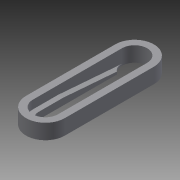
# Autodesk Inventor part: bed-holder
Saved by Autodesk Inventor 2015 (Build 190159000, 159)
## iProperties
Created: 2014-10-22
Part Number: bed-holder
Material: Generic
Document SubType Name: Modeling
Designer: caleb
Density: 1 g/cm^3
Appearance: Default
screw_diameter: 4.500 mm
screw_head_diameter: 7.500 mm
screw_head_clearance: 2.500 mm
wall: 2.000 mm
length: 38.000 mm
height: 4.500 mm
land_height: 2.000 mm
Author: caleb
Autodesk Inventor part; units mm, degrees
ref_plane "YZ Plane" through (0, 0, 0) normal (1, 0, 0) x (0, 1, 0)
ref_plane "XZ Plane" through (0, 0, 0) normal (0, 1, 0) x (-1, 0, 0)
ref_plane "XY Plane" through (0, 0, 0) normal (0, 0, 1) x (1, 0, 0)
sketch "Sketch6" plane through (0, 0, 0) normal (0, 0, 1) x (1, 0, 0)
  line L0 (0, 0) -> (0, -26.5) construction
  line L1 (-3.75, 0) -> (-3.75, -26.5)
  line L2 (3.75, -26.5) -> (3.75, 0)
  arc A0 (3.75, 0) -> (-3.75, 0) centre (0, 0) ccw
  arc A1 (-3.75, -26.5) -> (3.75, -26.5) centre (0, -26.5) ccw
  line L3 (5.75, 0) -> (5.75, -26.5)
  arc A2 (-5.75, -26.5) -> (5.75, -26.5) centre (0, -26.5) ccw
  line L4 (-5.75, -26.5) -> (-5.75, 0)
  arc A3 (5.75, 0) -> (-5.75, 0) centre (0, 0) ccw
  line L5 (0, 5.75) -> (0, -32.25) construction
  line L6 (0, 0) -> (0, -26.5) construction
  line L7 (-2.25, 0) -> (-2.25, -3)
  line L8 (2.25, -26.5) -> (2.25, -3)
  arc A4 (2.25, 0) -> (-2.25, 0) centre (0, 0) ccw
  arc A5 (-2.25, -26.5) -> (2.25, -26.5) centre (0, -26.5) ccw
  arc A6 (-3.75, 0) -> (3.75, 0) centre (0, 0) ccw
  line L9 (-2.25, -3) -> (-2.25, -26.5)
  line L10 (2.25, -3) -> (2.25, 0)
  point P0 (0, -13.25)
  point P1 (0, -13.25)
  dimension "d20" = 3.75
  dimension "d21" = 2
  dimension "d22" = 38
  dimension "d23" = 4.5
  constraints: 26 end point, 18 point on circle, 13 tangent, 7 centre point, 6 parallel, 2 midpoint, 1 collinear, 1 vertical, 3 other
  measures "d20" radius of A0
  measures "d21" distance between parallel lines of L3 L2
  measures "d22" distance of L5.start L5.end
  measures "d23" distance between parallel lines of L8 L7
extrude "Extrusion7" add sketch "Sketch6" along normal blind 4.5
sketch "Sketch7" plane through (0, 0, 0) normal (1, 0, 0) x (0, 1, 0)
  line L0 (0, 0.5) -> (-19, 2) construction
  line L1 (-19, 2) -> (-19, 0) construction
  point P0 (0, 0)
  point P1 (-26.5, 0)
  dimension "d28" = 7.5
  dimension "d29" = 2
  dimension "d30" = 0.5
  constraints: 4 end point, 1 horizontal alignment, 1 vertical, 1 vertical alignment
  measures "d28" horizontal distance of point (-26.5, 0) L0.end
  measures "d29" vertical distance of L0.end point (-26.5, 0)
  measures "d30" distance of point (0, 0) L0.start
ref_plane "Work Plane3" through (0, 0, 0.5) normal (0, 0.0787025, 0.9968981) x (0, -0.9968981, 0.0787025)
extrude "Extrusion9" add sketch "Sketch6" along normal blind 2 separate body contours A6 L9 A5 L8 L2 A1 L1
split "Split1" plane through (0, 0, 0.5) removes the side toward (0, 0.0787025, 0.9968981) bodies 2
combine bodies "Combine1" operation type add bodies to combine 1 2
equation "\"d20\" = 0.5 * screw_head_diameter"
equation "\"d21\" = wall"
equation "\"d22\" = length"
equation "\"d23\" = screw_diameter"
equation "\"d24\" = height"
equation "\"d28\" = screw_head_diameter"
equation "\"d29\" = land_height"
equation "\"d31\" = land_height"
equation "\"screw_diameter\" = 4.5"
equation "\"screw_head_diameter\" = 7.5"
equation "\"screw_head_clearance\" = 2.5"
equation "\"wall\" = 2"
equation "\"length\" = 38"
equation "\"height\" = land_height + screw_head_clearance"
equation "\"land_height\" = 2"
body "Solid2"
